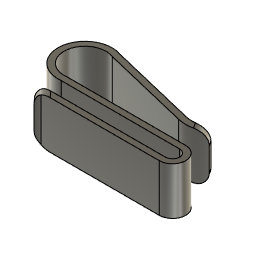
sunglass-clip (Autodesk Fusion 360 design; units mm, degrees)
Autodesk Fusion 360 part; units mm, degrees
sketch "Sketch1" plane through (0, 0, 0) normal (0, 0, 1) x (1, 0, 0)
  line L0 (0, 0) -> (-50, 0)
  arc A0 (-48.0531, 17) -> (-50, 0) centre (-51.318, 8.7624) ccw
  line L1 (-48.0531, 17) -> (-11.1134, 8.0861)
  arc A1 (-11.1134, 8.0861) -> (0.0968, 9.8611) centre (-7.6441, 22.4632) ccw
  line L2 (0.0968, 9.8611) -> (-1.3496, 11.9991)
  arc A2 (-10.5086, 10.5925) -> (-1.3496, 11.9991) centre (-7.6441, 22.4632) ccw
  line L3 (-11.1134, 8.0861) -> (-10.5086, 10.5925)
  line L4 (-10.5086, 10.5925) -> (-47.4483, 19.5064)
  line L5 (-47.4483, 19.5064) -> (-48.0531, 17)
  arc A3 (-47.4483, 19.5064) -> (-50, -2.5809) centre (-51.318, 8.7624) ccw
  line L6 (-50, 0) -> (-50, -2.5809)
  line L7 (-50, -2.5809) -> (0, -2.5809)
  line L8 (0, -2.5809) -> (0, 0)
  arc A4 (0, -8.5809) -> (0, -2.5809) centre (0, -5.5809) ccw
  line L9 (0, -8.5809) -> (-50, -8.5809)
  arc A5 (0, -11.1617) -> (0, 0) centre (0, -5.5809) ccw
  line L10 (0, -8.5809) -> (0, -11.1617)
  line L11 (0, -11.1617) -> (-50, -11.1617)
  arc A6 (-50, -11.1617) -> (-52.2756, -11.8049) centre (-50, -15.5093) ccw
  arc A7 (-50, -8.5809) -> (-54.0353, -9.8773) centre (-50, -15.5093) ccw
  line L12 (-52.2756, -11.8049) -> (-54.0353, -9.8773)
  dimension "d1" = 50
  dimension "d2" = 17
  dimension "d3" = 38
  dimension "d4" = 50
  dimension "d5" = 3
  dimension "d6" = 50
  constraint coincident L0.start L8.end
  constraint horizontal L0
  constraint tangent L1 A1
  constraint coincident A1.centre A2.centre
  constraint perpendicular L1 L3
  constraint tangent A2 L4
  constraint perpendicular L1 L5
  constraint coincident A0.centre A3.centre
  constraint perpendicular L0 L6
  constraint perpendicular L6 L7
  constraint perpendicular L7 L8
  constraint tangent L7 A4
  constraint tangent A4 L9
  constraint parallel L0 L9
  constraint coincident A4.centre A5.centre
  constraint vertical L10
  constraint tangent A5 L11
  constraint tangent L11 A6
  constraint coincident A6.centre A7.centre
  measures "d1" horizontal distance of L0.start L0.end
  measures "d2" vertical distance of L0.end A0.start
  measures "d3" distance of A0.start L1.end
  measures "d4" horizontal distance of A4.start L9.end
  measures "d5" vertical distance of L7.end A4.centre
  measures "d6" horizontal distance of A5.start L11.end
extrude "Extrude1" add sketch "Sketch1" along normal blind 20
fillet "Fillet1" radius 5 2 edges at (-53.1554, -10.8411, 20) (-53.1554, -10.8411, 0)
fillet "Fillet2" radius 5 2 edges at (-0.6264, 10.9301, 0) (-0.6264, 10.9301, 20)
